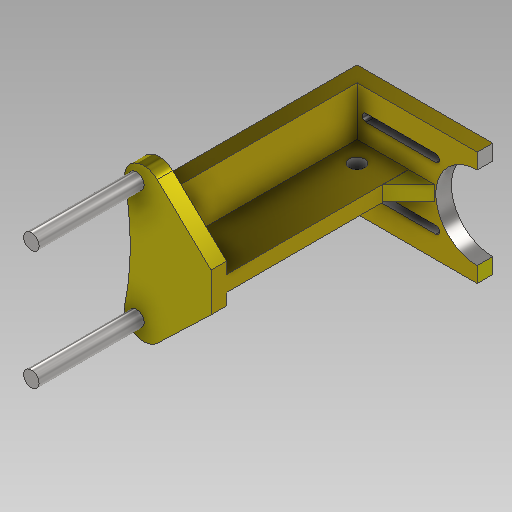
# Autodesk Inventor part: garra_griper
Saved by Autodesk Inventor 2021 (Build 250183000, 183)
## iProperties
Created: 2022-01-31
Part Number: garra_griper
Material: Acerito
Document SubType Name: Modeling
Designer: edibe
Density: 8 g/cm^3
Appearance: Semipulido
Mass: 48132.2 g
Surface Area: 4977.51 cm^2
Volume: 6016.52 cm^3
Author: edibe
Autodesk Inventor part; units mm, degrees
ref_plane "YZ Plane" through (0, 0, 0) normal (1, 0, 0) x (0, 1, 0)
ref_plane "XZ Plane" through (0, 0, 0) normal (0, 1, 0) x (-1, 0, 0)
ref_plane "XY Plane" through (0, 0, 0) normal (0, 0, 1) x (1, 0, 0)
sketch "Boceto7" plane through (0, 0, 0) normal (0, 0, 1) x (1, 0, 0)
  circle A0 centre (0, 0) radius 330 construction
  line L0 (-311.127, 110) -> (311.127, 110)
  line L1 (311.127, 110) -> (311.127, -110)
  line L2 (311.127, -110) -> (-311.127, -110)
  line L3 (-311.127, -110) -> (-311.127, 110)
  line L4 (-311.127, 110) -> (311.127, -110) construction
  line L5 (311.127, 110) -> (-311.127, -110) construction
  dimension "d23" = 660
  dimension "d24" = 220
  constraints: 12 end point, 2 coincident, 2 parallel, 2 point on circle, 1 centre point, 1 horizontal, 1 midpoint, 1 perpendicular
  measures "d23" diameter of A0
  measures "d24" distance between parallel lines of L2 L0
extrude "Extrusión4" add sketch "Boceto7" along normal blind 30
sketch "Boceto8" plane through (0, 0, 30) normal (0, 0, 1) x (1, 0, 0)
  line L0 (311.127, 110) -> (-311.127, 110) projected
  line L1 (-311.127, -110) -> (311.127, -110) projected
  line L2 (-311.127, 110) -> (-281.127, 110)
  line L3 (-281.127, 110) -> (-281.127, -110)
  line L4 (-281.127, -110) -> (-311.127, -110)
  line L5 (-311.127, -110) -> (-311.127, 110)
  line L6 (-281.127, -15) -> (-181.127, -15)
  line L7 (-181.127, -15) -> (-181.127, 15)
  line L8 (-181.127, 15) -> (-281.127, 15)
  line L9 (-281.127, 15) -> (-281.127, -15)
  point P0 (0, 0)
  point P1 (-281.127, 0)
  dimension "d27" = 30
  dimension "d29" = 30
  dimension "d32" = 100
  constraints: 16 end point, 4 parallel, 2 horizontal, 2 midpoint, 2 perpendicular, 1 point on line
  measures "d27" distance between parallel lines of L5 L3
  measures "d29" distance of L6.end L7.end
  measures "d32" distance of L6.start L6.end
extrude "Extrusión5" add sketch "Boceto8" along normal blind 352.3
sketch "Boceto14" plane through (0, 0, 382.3) normal (0, 0, 1) x (1, 0, 0)
  line L0 (-311.127, 110) -> (-311.127, -110) projected
  circle A0 centre (-311.127, 110) radius 30 construction
  circle A1 centre (-325.2691, 115) radius 15 construction
  circle A2 centre (0, 0) radius 330 construction
  line L1 (-181.127, 37.5) -> (-181.127, -37.5)
  line L2 (-181.127, -15) -> (-181.127, 15) projected
  circle A3 centre (-311.127, -110) radius 30 construction
  circle A4 centre (-325.2691, -115) radius 15 construction
  arc A5 (-347.8333, -102.3256) -> (-347.8333, 102.3256) centre (-837.2508, 0) ccw
  line L3 (-181.127, -37.5) -> (-285.2, -137.0932)
  line L4 (-181.127, 37.5) -> (-285.2, 137.0932)
  arc A6 (-285.2, 137.0932) -> (-347.8333, 102.3256) centre (-311.127, 110) ccw
  arc A7 (-347.8333, -102.3256) -> (-285.2, -137.0932) centre (-311.127, -110) ccw
  point P0 (-181.127, 0)
  dimension "d61" = 60
  dimension "d62" = 660
  dimension "d63" = 75
  dimension "d64" = 60
  dimension "d65" = 30
  dimension "d66" = 30
  dimension "d69" = 1000
  constraints: 8 centre point, 6 end point, 6 point on circle, 6 tangent, 5 coincident, 2 midpoint, 1 vertical
  measures "d61" diameter of A0
  measures "d62" diameter of A2
  measures "d63" distance of L1.start L1.end
  measures "d64" diameter of A3
  measures "d65" diameter of A4
  measures "d66" diameter of A1
  measures "d69" diameter of A5
extrude "Extrusión8" add sketch "Boceto14" along normal blind 30
sketch "Boceto15" plane through (0, 0, 412.3) normal (0, 0, 1) x (1, 0, 0)
  circle A0 centre (0, 0) radius 330 construction
  line L0 (-311.127, 110) -> (-311.127, -110) projected
  line L1 (311.127, 110) -> (-311.127, 110) projected
  circle A1 centre (-311.127, 110) radius 30 construction
  circle A2 centre (-325.2691, 115) radius 15
  circle A3 centre (-311.127, -110) radius 30 construction
  circle A4 centre (-325.2691, -115) radius 15
  dimension "d72" = 660
  dimension "d73" = 60
  dimension "d74" = 30
  dimension "d75" = 60
  dimension "d76" = 30
  constraints: 5 centre point, 4 tangent, 3 coincident
  measures "d72" diameter of A0
  measures "d73" diameter of A1
  measures "d74" diameter of A2
  measures "d75" diameter of A3
  measures "d76" diameter of A4
extrude "Extrusión9" add sketch "Boceto15" along normal blind 203.25
ref_plane "Plano de trabajo2" through (-281.127, 0, 30) normal (0, -1, 0) x (1, 0, 0)
sketch "Boceto16" plane through (-281.127, 0, 30) normal (0, -1, 0) x (1, 0, 0)
  line L0 (100, 50) -> (150, 0)
  point P0 (281.127, -30)
  point P1 (562.254, 0)
  constraints: 2 end point
extrude "Nervio1" add sketch "Boceto16" along normal mid plane 29 rib yes fills toward (124.9646, 24.9646) open curves L0
sketch "Boceto18" plane through (0, 0, 30) normal (0, 0, 1) x (1, 0, 0)
  line L0 (311.127, -110) -> (311.127, 110) projected
  line L1 (311.127, 110) -> (-281.127, 110) construction
  line L2 (311.127, -110) -> (-48.873, -110)
  line L3 (-48.873, -110) -> (-48.873, 110)
  line L4 (-48.873, 110) -> (311.127, 110)
  line L5 (311.127, 110) -> (311.127, -110)
  arc A0 (-48.873, 80) -> (-48.873, -80) centre (-48.873, 0) ccw
  point P0 (0, 0)
  dimension "d114" = 360
  dimension "d115" = 160
  constraints: 8 end point, 3 point on line, 2 parallel, 2 point on circle, 1 centre point, 1 horizontal, 1 midpoint, 1 perpendicular
  measures "d114" distance between parallel lines of L0 L3
  measures "d115" diameter of A0
extrude "Extrusión10" cut sketch "Boceto18" against normal through all
sketch "Boceto19" plane through (0, 0, 30) normal (0, 0, 1) x (1, 0, 0)
  line L0 (-263.873, 67.5) -> (-128.873, 67.5)
  line L1 (-121.373, 60) -> (-121.373, 60)
  line L2 (-128.873, 52.5) -> (-263.873, 52.5)
  line L3 (-271.373, 60) -> (-271.373, 60)
  line L4 (-48.873, 110) -> (-281.127, 110) projected
  arc A0 (-271.373, 60) -> (-263.873, 52.5) centre (-263.873, 60) ccw
  arc A1 (-263.873, 67.5) -> (-271.373, 60) centre (-263.873, 60) ccw
  arc A2 (-121.373, 60) -> (-128.873, 67.5) centre (-128.873, 60) ccw
  arc A3 (-128.873, 52.5) -> (-121.373, 60) centre (-128.873, 60) ccw
  line L5 (-48.873, -110) -> (-48.873, 110) projected
  point P0 (0, 0)
  point P1 (-271.373, 67.5)
  point P2 (-121.373, 67.5)
  dimension "d101" = 150
  dimension "d102" = 15
  dimension "d104" = 7.5
  dimension "d105" = 80
  dimension "d113" = 50
  constraints: 8 end point, 8 point on circle, 8 tangent, 4 centre point, 4 point on line, 3 equal radius, 2 parallel, 1 horizontal, 1 perpendicular, 1 other
  measures "d101" distance of point (-271.373, 67.5) point (-121.373, 67.5)
  measures "d102" distance between parallel lines of L0 L2
  measures "d104" radius of A0
  measures "d113" distance from line of L4 A2.centre
extrude "Extrusión11" cut sketch "Boceto19" against normal through all
mirror "Simetría1" about plane through (0, 0, 0) normal (0, 1, 0) of "Extrusión11"
sketch "Boceto20" plane through (-281.127, 15, 30) normal (0, 1, 0) x (1, 0, 0)
  circle A0 centre (40, -40) radius 15
  line L0 (0, 0) -> (0, -352.3) projected
  line L1 (232.254, 0) -> (0, 0) projected
  point P0 (281.127, 30)
  dimension "d108" = 30
  dimension "d109" = 40
  dimension "d110" = 40
  constraints: 1 centre point
  measures "d108" diameter of A0
  measures "d109" distance from line of L0 A0.centre
  measures "d110" distance from line of L1 A0.centre
extrude "Extrusión12" cut sketch "Boceto20" against normal through all
equation "\"d23\" = diametro_llanta"
equation "\"d24\" = 0.333333 * diametro_llanta"
equation "\"d25\" = espesor_soporte"
equation "\"d27\" = espesor_soporte"
equation "\"d29\" = espesor_soporte"
equation "\"d35\" = 1.3 * ancho_llanta"
equation "\"d61\" = 2 * diametro_tubo_garrita"
equation "\"d62\" = diametro_llanta"
equation "\"d63\" = 2.5 * espesor_soporte"
equation "\"d64\" = 2 * diametro_tubo_garrita"
equation "\"d65\" = diametro_tubo_garrita"
equation "\"d66\" = diametro_tubo_garrita"
equation "\"d70\" = espesor_soporte"
equation "\"d72\" = diametro_llanta"
equation "\"d73\" = 2 * diametro_tubo_garrita"
equation "\"d74\" = diametro_tubo_garrita"
equation "\"d75\" = 2 * diametro_tubo_garrita"
equation "\"d76\" = diametro_tubo_garrita"
equation "\"d77\" = 0.75 * ancho_llanta"
equation "\"d102\" = 0.5 * espesor_soporte"
equation "\"d108\" = espesor_soporte"
equation "\"diametro_llanta\" = 660"
equation "\"ancho_llanta\" = 271"
equation "\"espesor_soporte\" = 30"
equation "\"diametro_tubo_garrita\" = 30"
equation "\"d67\" = 2.5 * diametro_tubo_garrita"
equation "\"d68\" = 2.5 * diametro_tubo_garrita"
